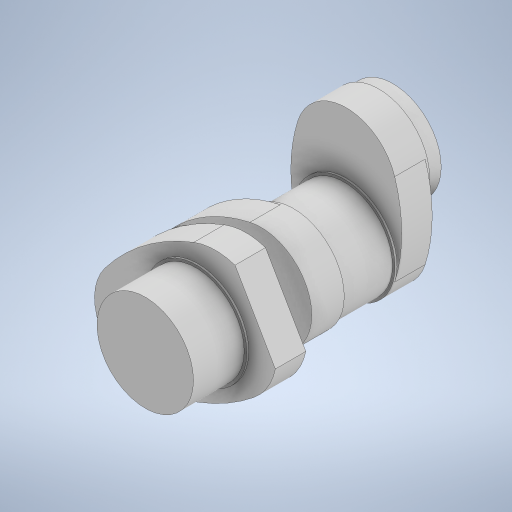
# Autodesk Inventor part: Malec Klika_ok
Saved by Autodesk Inventor 2024 (Build 280153020, 153B)
## iProperties
Created: 2024-06-06
Part Number: Malec Klika_ok
Material: Všeobecné
Document SubType Name: Modeling
Designer: malecdaniel
Density: 1 g/cm^3
Appearance: Výchozí
Author: malecdaniel
Autodesk Inventor part; units mm, degrees
ref_plane "YZ Plane" through (0, 0, 0) normal (1, 0, 0) x (0, 1, 0)
ref_plane "XZ Plane" through (0, 0, 0) normal (0, 1, 0) x (-1, 0, 0)
ref_plane "XY Plane" through (0, 0, 0) normal (0, 0, 1) x (1, 0, 0)
sketch "Sketch8" plane through (0, 0, 0) normal (0, 0, 1) x (1, 0, 0)
  circle A0 centre (-33.5564, 13.121) radius 47.5
  point P0 (0, 0)
  dimension "d28" = 95
  constraints: 1 centre point
  measures "d28" diameter of A0
extrude "Extrusion6" add sketch "Sketch8" along normal blind 14
sketch "Sketch9" plane through (-33.5564, 13.121, 14) normal (0, 0, 1) x (1, 0, 0)
  circle A0 centre (0, 0) radius 50
  point P0 (33.5564, -13.121)
  dimension "d31" = 100
  constraints: 1 centre point
  measures "d31" diameter of A0
extrude "Extrusion7" add sketch "Sketch9" along normal blind 2
sketch "Sketch10" plane through (-33.5564, 13.121, 16) normal (0, 0, 1) x (1, 0, 0)
  circle A0 centre (0, 0) radius 50 projected
  arc A1 (-47.697, -75) -> (47.697, -75) centre (0, -60) ccw
  arc A2 (47.697, 15) -> (-47.697, 15) centre (0, 0) ccw
  line L0 (-61.4591, 15) -> (62.8598, 15) construction
  arc A3 (47.697, -75) -> (47.697, 15) centre (-95.3939, -30) ccw
  line L1 (0, 0) -> (0, -112.0986) construction
  arc A4 (-47.697, 15) -> (-47.697, -75) centre (95.3939, -30) ccw
  point P0 (33.5564, -13.121)
  point P1 (47.697, 15)
  point P2 (-47.697, 15)
  dimension "d34" = 100
  dimension "d35" = 60
  dimension "d37" = 100
  dimension "d38" = 150
  constraints: 8 point on circle, 4 centre point, 4 end point, 3 point on line, 2 symmetric about line, 2 tangent, 1 coincident, 1 horizontal, 1 vertical, 1 other
  measures "d34" diameter of A1
  measures "d35" distance of A1.centre A0.centre
  measures "d37" diameter of A2
  measures "d38" radius of A3
extrude "Extrusion8" add sketch "Sketch10" along normal blind 30
sketch "Sketch15" plane through (-33.5564, 13.121, 46) normal (0, 0, 1) x (1, 0, 0)
  circle A0 centre (0, 0) radius 47.5 projected
  circle A1 centre (0, 0) radius 47.5 projected
  line L0 (0, 0) -> (0, -60)
  circle A2 centre (0, -60) radius 50
  point P0 (33.5564, -13.121)
  dimension "d61" = 60
  dimension "d62" = 100
  constraints: 2 end point, 1 centre point, 1 coincident, 1 vertical
  measures "d61" distance of L0.start L0.end
  measures "d62" diameter of A2
extrude "Extrusion13" add sketch "Sketch15" along normal blind 2 contours A2 L0 A0 | A0 A2 | A0 L0 A2 picked at (-1.9859, -88.9539)
sketch "Sketch16" plane through (-33.5564, -46.879, 48) normal (0, 0, 1) x (1, 0, 0)
  circle A0 centre (0, 0) radius 47.5
  point P0 (33.5564, 46.879)
  dimension "d65" = 95
  constraints: 1 centre point
  measures "d65" diameter of A0
extrude "Extrusion14" add sketch "Sketch16" along normal blind 50
sketch "Sketch22" plane through (-33.5564, -46.879, 98) normal (0, 0, 1) x (1, 0, 0)
  circle A0 centre (0, 0) radius 50
  point P0 (33.5564, 46.879)
  dimension "d92" = 100
  constraints: 1 centre point
  measures "d92" diameter of A0
extrude "Extrusion20" add sketch "Sketch22" along normal blind 2
sketch "Sketch23" plane through (-33.5564, -46.879, 100) normal (0, 0, 1) x (1, 0, 0)
  line L0 (0, 0) -> (0, 136.4462) construction
  line L1 (0, 0) -> (-102.7311, -59.3118) construction
  line L2 (0, 0) -> (-51.9615, -30) construction
  arc A0 (-88.8004, 3.8068) -> (-41.1034, -78.8068) centre (-51.9615, -30) ccw
  arc A1 (-10.8581, 48.8068) -> (-88.8004, 3.8068) centre (21.7162, -97.6136) ccw
  arc A2 (-41.1034, -78.8068) -> (36.8389, -33.8068) centre (-73.6777, 67.6136) ccw
  arc A3 (36.8389, -33.8068) -> (-10.8581, 48.8068) centre (0, 0) ccw
  circle A4 centre (0, 0) radius 50 projected
  point P0 (33.5564, 46.879)
  dimension "d95" = 120
  dimension "d96" = 60
  dimension "d101" = 150
  constraints: 10 point on circle, 6 end point, 4 centre point, 4 tangent, 2 coincident, 2 equal radius, 1 concentric, 1 point on line, 1 vertical
  measures "d95" angle of L0 L1
  measures "d96" distance of L0.start L2.end
  measures "d101" radius of A2
extrude "Extrusion21" add sketch "Sketch23" along normal blind 30
sketch "Sketch31" plane through (-33.5564, -46.879, 130) normal (0, 0, 1) x (1, 0, 0)
  arc A0 (-88.8004, 3.8068) -> (-41.1034, -78.8068) centre (-51.9615, -30) ccw projected
  circle A1 centre (-51.9615, -30) radius 50
  point P0 (33.5564, 46.879)
  point P1 (-41.1034, -78.8068)
  point P2 (-88.8004, 3.8068)
  dimension "d144" = 100
  constraints: 1 centre point, 1 coincident
  measures "d144" diameter of A1
extrude "Extrusion29" add sketch "Sketch31" along normal blind 2
sketch "Sketch32" plane through (-85.5179, -76.879, 132) normal (0, 0, 1) x (1, 0, 0)
  circle A0 centre (0, 0) radius 47.5
  point P0 (85.5179, 76.879)
  dimension "d147" = 95
  constraints: 1 centre point
  measures "d147" diameter of A0
extrude "Extrusion30" add sketch "Sketch32" along normal blind 28
sketch "Sketch33" plane through (-85.5179, -76.879, 160) normal (0, 0, 1) x (1, 0, 0)
  circle A0 centre (0, 0) radius 50
  point P0 (85.5179, 76.879)
  dimension "d150" = 100
  constraints: 1 centre point
  measures "d150" diameter of A0
extrude "Extrusion31" add sketch "Sketch33" along normal blind 2
sketch "Sketch34" plane through (-85.5179, -76.879, 162) normal (0, 0, 1) x (1, 0, 0)
  line L0 (0, 0) -> (134.2711, 77.5215) construction
  line L1 (0, 0) -> (155.0429, 0) construction
  line L2 (0, 0) -> (69.282, 40) construction
  arc A0 (-39.826, 30.2306) -> (6.2675, -49.6056) centre (0, 0) ccw
  line L3 (73.1921, 123.2275) -> (151.6531, -12.6708)
  arc A1 (47.7695, 96.0108) -> (-39.826, 30.2306) centre (119.478, -90.6919) ccw
  circle A2 centre (0, 0) radius 50 projected
  arc A3 (107.0325, -6.6358) -> (128.0963, 28.1307) centre (69.282, 40) ccw
  arc A4 (88.41, 96.8693) -> (47.7695, 96.0108) centre (69.282, 40) ccw
  arc A5 (6.2675, -49.6056) -> (107.0325, -6.6358) centre (-18.8025, 148.8169) ccw
  point P0 (85.5179, 76.879)
  dimension "d153" = 30
  dimension "d155" = 80
  dimension "d158" = 125
  dimension "d159" = 60
  dimension "d160" = 200
  constraints: 12 point on circle, 8 end point, 5 centre point, 4 tangent, 3 point on line, 2 coincident, 2 equal radius, 1 concentric, 1 equal length, 1 horizontal, 1 perpendicular
  measures "d153" angle of L1 L0
  measures "d155" distance of L0.start L2.end
  measures "d158" distance from line of L0.start L3
  measures "d159" radius of A4
  measures "d160" radius of A1
extrude "Extrusion32" add sketch "Sketch34" along normal blind 30
sketch "Sketch35" plane through (-85.5179, -76.879, 192) normal (0, 0, 1) x (1, 0, 0)
  circle A0 centre (51.9615, 30) radius 47.5 projected
  circle A1 centre (51.9615, 30) radius 50
  point P0 (85.5179, 76.879)
  dimension "d163" = 100
  constraints: 1 centre point, 1 coincident
  measures "d163" diameter of A1
extrude "Extrusion33" add sketch "Sketch35" along normal blind 2 contours A0 | A1
sketch "Sketch36" plane through (-33.5564, -46.879, 194) normal (0, 0, 1) x (1, 0, 0)
  circle A0 centre (0, 0) radius 47.5
  point P0 (33.5564, 46.879)
  dimension "d166" = 95
  constraints: 1 centre point
  measures "d166" diameter of A0
extrude "Extrusion34" add sketch "Sketch36" along normal blind 50
body "Solid4"
